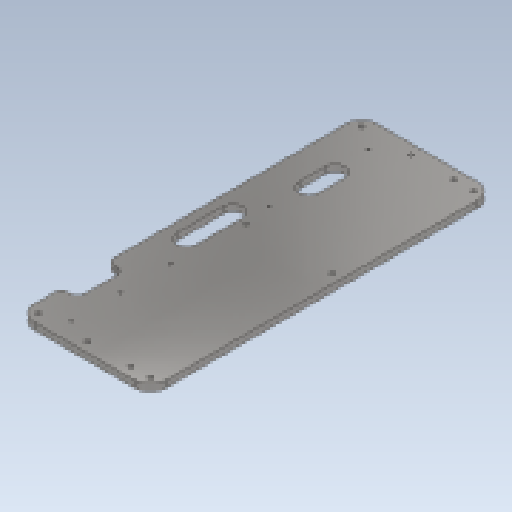
# Autodesk Inventor part: Current_plate
Saved by Autodesk Inventor 2025.2 (Build 292293000, 293)
## iProperties
Created: 2025-02-20
Part Number: Current_plate
Material: Stainless Steel
Document SubType Name: Modeling
Designer: Sergio Quintero
Density: 8 g/cm^3
Appearance: Semi-Polished
Mass: 8245.1 g
Surface Area: 2223.4 cm^2
Volume: 1030.64 cm^3
Author: Sergio Quintero
Autodesk Inventor part; units mm, degrees
note: some values were not read from the file. Chosen so that the rebuilt part matches the saved one: pattern direction of "Rectangular Pattern1".
ref_plane "YZ Plane" through (0, 0, 0) normal (1, 0, 0) x (0, 1, 0)
ref_plane "XZ Plane" through (0, 0, 0) normal (0, 1, 0) x (-1, 0, 0)
ref_plane "XY Plane" through (0, 0, 0) normal (0, 0, 1) x (1, 0, 0)
sketch "Sketch1" plane through (0, 0, 0) normal (0, 1, 0) x (-1, 0, 0)
  line L0 (-100, -260) -> (100, -260)
  line L1 (100, -260) -> (100, 260)
  line L2 (100, 260) -> (-100, 260)
  line L3 (-100, 260) -> (-100, -260)
  line L4 (-100, -260) -> (100, 260) construction
  line L5 (100, -260) -> (-100, 260) construction
  point P0 (0, 0)
  dimension "d0" = 200
  dimension "d1" = 520
  constraints: 12 end point, 2 midpoint, 2 parallel, 1 horizontal, 1 perpendicular
  measures "d0" distance of L2.end L1.end
  measures "d1" distance of L1.end L0.end
extrude "Extrusion1" add sketch "Sketch1" along normal blind 10
fillet "Fillet1" radius 25 4 edges at (-100, 5, -260) (-100, 5, 260) (100, 5, 260) (100, 5, -260)
sketch "Sketch2" plane through (0, 10, 0) normal (0, 1, 0) x (1, 0, 0)
  line L0 (100, -235) -> (100, 235) projected
  line L1 (-75, -260) -> (75, -260) projected
  point P0 (0, 0)
  point P1 (85, -245)
  dimension "d5" = 15
  dimension "d6" = 15
  measures "d5" distance from line of L0 point (85, -245)
  measures "d6" distance from line of point (85, -245) L1
hole "Hole1" at (85, 10, 245) direction (0, -1, 0) diameter 6.647 end through all thread size "M8x1.25" class "6H" standard "ISO Metric profile"
pattern_linear "Rectangular Pattern1" count 2 spacing 170 along (-1, 0, 0) count 2 spacing 490 along (0, 0, -1) of "Hole1"
sketch "Sketch3" plane through (0, 10, 0) normal (0, 1, 0) x (1, 0, 0)
  line L0 (-75, -260) -> (75, -260) projected
  line L1 (-100, 235) -> (-100, -235) projected
  point P0 (0, 0)
  point P1 (-10, -245)
  point P2 (55, -245)
  dimension "d20" = 15
  dimension "d21" = 90
  dimension "d22" = 65
  dimension "d23" = 15
  measures "d20" distance from line of L0 point (-10, -245)
  measures "d21" distance from line of L1 point (-10, -245)
  measures "d22" distance of point (-10, -245) point (55, -245)
  measures "d23" distance from line of L0 point (55, -245)
hole "Hole2" at (-10, 10, 245) at (55, 10, 245) direction (0, -1, 0) diameter 6.647 end through all thread size "M8x1.25" class "6H" standard "ISO Metric profile"
mirror "Mirror1" about plane through (0, 0, 0) normal (0, 0, 1) of "Hole2"
sketch "Sketch4" plane through (0, 10, 0) normal (0, 1, 0) x (1, 0, 0)
  line L0 (75, 260) -> (-75, 260) projected
  line L1 (100, -235) -> (100, 235) projected
  point P0 (0, 0)
  point P1 (-45, 30)
  point P2 (85, 30)
  dimension "d31" = 230
  dimension "d32" = 145
  dimension "d33" = 230
  dimension "d34" = 15
  measures "d31" distance from line of L0 point (-45, 30)
  measures "d32" distance from line of L1 point (-45, 30)
  measures "d33" distance from line of L0 point (85, 30)
  measures "d34" distance from line of L1 point (85, 30)
hole "Hole3" at (-45, 10, -30) at (85, 10, -30) direction (0, -1, 0) diameter 6.647 end through all thread size "M8x1.25" class "6H" standard "ISO Metric profile"
sketch "Sketch8" plane through (0, 10, 0) normal (0, 1, 0) x (1, 0, 0)
  line L0 (-100, 235) -> (-100, -235) projected
  line L1 (-100, -125) -> (-75, -125)
  line L2 (-75, -125) -> (-75, -195)
  line L3 (-75, -195) -> (-100, -195)
  line L4 (-100, -195) -> (-100, -125)
  line L5 (-75, -260) -> (75, -260) projected
  point P0 (0, 0)
  dimension "d72" = 25
  dimension "d73" = 70
  dimension "d74" = 65
  constraints: 8 end point, 2 parallel, 1 horizontal, 1 perpendicular, 1 point on line
  measures "d72" distance of L2.end L3.end
  measures "d73" distance of L1.end L2.end
  measures "d74" distance between parallel lines of L5 L3
extrude "Extrusion2" cut sketch "Sketch8" against normal blind 10
fillet "Fillet2" radius 10 4 edges at (-100, 5, 125) (-75, 5, 125) (-100, 5, 195) (-75, 5, 195)
sketch "Sketch9" plane through (0, 10, 0) normal (0, 1, 0) x (1, 0, 0)
  line L0 (-55, 50) -> (-85, 50)
  line L1 (-85, 50) -> (-85, -50)
  line L2 (-85, -50) -> (-55, -50)
  line L3 (-55, -50) -> (-55, 50)
  line L4 (-100, 235) -> (-100, -115) projected
  line L5 (75, 260) -> (-75, 260) projected
  point P0 (0, 0)
  dimension "d78" = 30
  dimension "d79" = 100
  dimension "d80" = 15
  dimension "d81" = 210
  constraints: 8 end point, 2 parallel, 1 horizontal, 1 perpendicular
  measures "d78" distance of L2.end L1.end
  measures "d79" distance of L1.end L0.end
  measures "d80" distance between parallel lines of L4 L1
  measures "d81" distance between parallel lines of L0 L5
extrude "Extrusion3" cut sketch "Sketch9" against normal blind 10
fillet "Fillet3" radius 15 4 edges at (-55, 5, -50) (-55, 5, 50) (-85, 5, 50) (-85, 5, -50)
sketch "Sketch10" plane through (0, 10, 0) normal (0, 1, 0) x (1, 0, 0)
  line L0 (-30, 180) -> (-60, 180)
  line L1 (-60, 180) -> (-60, 110)
  line L2 (-60, 110) -> (-30, 110)
  line L3 (-30, 110) -> (-30, 180)
  line L4 (-100, 235) -> (-100, -115) projected
  line L5 (75, 260) -> (-75, 260) projected
  point P0 (0, 0)
  dimension "d85" = 30
  dimension "d86" = 70
  dimension "d87" = 40
  dimension "d88" = 80
  constraints: 8 end point, 2 parallel, 1 horizontal, 1 perpendicular
  measures "d85" distance of L2.end L1.end
  measures "d86" distance of L1.end L0.end
  measures "d87" distance between parallel lines of L4 L1
  measures "d88" distance between parallel lines of L5 L0
extrude "Extrusion4" cut sketch "Sketch10" against normal blind 10
fillet "Fillet4" radius 15 4 edges at (-60, 5, -110) (-60, 5, -180) (-30, 5, -180) (-30, 5, -110)
sketch "Sketch11" plane through (0, 10, 0) normal (0, 1, 0) x (1, 0, 0)
  line L0 (-100, 235) -> (-100, -115) projected
  line L1 (-100, -205) -> (-100, -235) projected
  line L2 (75, 260) -> (-75, 260) projected
  line L3 (-75, -260) -> (75, -260) projected
  point P0 (0, 0)
  point P1 (-50, 220)
  point P2 (-50, 70)
  point P3 (-50, -80)
  point P4 (-50, -155)
  point P5 (-50, -230)
  dimension "d92" = 50
  dimension "d93" = 50
  dimension "d94" = 50
  dimension "d95" = 50
  dimension "d96" = 50
  dimension "d97" = 40
  dimension "d98" = 190
  dimension "d99" = 180
  dimension "d100" = 105
  dimension "d101" = 30
  measures "d92" distance from line of L0 point (-50, 220)
  measures "d93" distance from line of L0 point (-50, 70)
  measures "d94" distance from line of L0 point (-50, -80)
  measures "d95" distance from line of L0 point (-50, -155)
  measures "d96" distance from line of L1 point (-50, -230)
  measures "d97" distance from line of L2 point (-50, 220)
  measures "d98" distance from line of L2 point (-50, 70)
  measures "d99" distance from line of L3 point (-50, -80)
  measures "d100" distance from line of L3 point (-50, -155)
  measures "d101" distance from line of L3 point (-50, -230)
hole "Hole7" at (-50, 10, -220) at (-50, 10, -70) at (-50, 10, 80) at (-50, 10, 155) at (-50, 10, 230) direction (0, -1, 0) diameter 4.134 end through all thread size "M5x0.8" class "6H" standard "ISO Metric profile"
body "Solid1"
